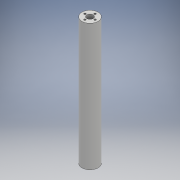
# Autodesk Inventor part: barra solida hueca para imprimir 3D
Saved by Autodesk Inventor 2018 (Build 220112000, 112)
## iProperties
Created: 2019-05-18
Part Number: barra solida hueca para imprimir 3D
Material: Generic
Document SubType Name: Modeling
Designer: JLVega003
Density: 1 g/cm^3
Appearance: Default
Author: JLVega003
Autodesk Inventor part; units mm, degrees
ref_plane "YZ Plane" through (0, 0, 0) normal (1, 0, 0) x (0, 1, 0)
ref_plane "XZ Plane" through (0, 0, 0) normal (0, 1, 0) x (-1, 0, 0)
sketch "Sketch1" plane through (0, 0, 0) normal (0, 0, 1) x (1, 0, 0)
  circle A0 centre (0, 0) radius 12.7
  circle A1 centre (0, 0) radius 5
  dimension "d0" = 25.4
  dimension "d1" = 10
  constraints: 2 centre point, 2 coincident
  measures "d0" diameter of A0
  measures "d1" diameter of A1
extrude "Extrusion1" add sketch "Sketch1" along normal mid plane 200
sketch "Sketch2" plane through (0, 0, 100) normal (0, 0, 1) x (1, 0, 0)
  line L0 (-17.78, 0) -> (17.78, 0) projected
  line L1 (0, -17.78) -> (0, 17.78) projected
  circle A0 centre (0, 0) radius 8 construction
  line L2 (0, 0) -> (8, 0) construction
  circle A1 centre (0, 8) radius 1.5
  circle A2 centre (-8, 0) radius 1.5
  circle A3 centre (0, -8) radius 1.5
  circle A4 centre (8, 0) radius 1.5
  point P0 (8, 0)
  point P1 (0, -8)
  point P2 (-8, 0)
  dimension "d4" = 16
  dimension "d25" = 3
  dimension "d28" = 360
  constraints: 5 centre point, 4 point on circle, 4 point on line, 3 coincident, 2 end point, 1 horizontal, 9 other
  measures "d4" diameter of A0
  measures "d25" diameter of A1
extrude "Extrusion3" cut sketch "Sketch2" against normal blind 15
thread "Thread1" size "M3x0.5" class "6H" standard "ANSI Metric M Profile" full length
thread "Thread2" size "M3x0.5" class "6H" standard "ANSI Metric M Profile" full length
thread "Thread3" size "M3x0.5" class "6H" standard "ANSI Metric M Profile" full length
thread "Thread4" size "M3x0.5" class "6H" standard "ANSI Metric M Profile" full length
mirror "Mirror2" about plane through (0, 0, 0) normal (0, 0, 1) of "Extrusion3"
thread "Thread5" size "M3x0.5" class "6H" standard "ANSI Metric M Profile" full length
thread "Thread6" size "M3x0.5" class "6H" standard "ANSI Metric M Profile" full length
thread "Thread7" size "M3x0.5" class "6H" standard "ANSI Metric M Profile" full length
thread "Thread8" size "M3x0.5" class "6H" standard "ANSI Metric M Profile" full length
ref_plane "Work Plane1" through (0, 0, -80) normal (0, 0, -1) x (-1, 0, 0)
sketch "Sketch3" plane through (0, 0, -80) normal (0, 0, -1) x (-1, 0, 0)
  circle A0 centre (0, 0) radius 7.9375
  dimension "d49" = 15.875
  constraints: 1 centre point, 1 coincident
  measures "d49" diameter of A0
extrude "Extrusion4" cut sketch "Sketch3" against normal blind 160
chamfer "Chamfer3" distance 2.9375 angle 45 2 edges at (7.9375, 0, 80) (7.9375, 0, -80)
body "Solid1"
